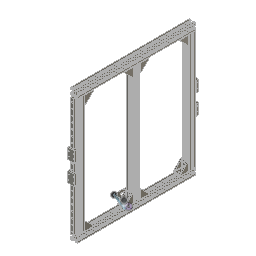
сборка станка вер 1.1.1 (Autodesk Fusion 360 design; units mm, degrees)
Autodesk Fusion 360 part; units mm, degrees
sketch "Sketch1" plane through (0, 0, 0) normal (0, 1, 0) x (1, 0, 0)
  line L0 (6.0101, -7) -> (-6.0101, -7)
  line L1 (-8.1, -12.8) -> (-8.1, -9.0899)
  line L2 (-6.0101, -7) -> (-8.1, -9.0899)
  line L3 (-4.1, -14.2) -> (-4.9, -14.2)
  line L4 (-4.9, -14.2) -> (-4.9, -15)
  line L5 (-4.1, -14.2) -> (-4.1, -12.8)
  line L6 (-13, -15) -> (-4.9, -15)
  line L7 (-8.1, -12.8) -> (-4.1, -12.8)
  line L8 (6.0101, -7) -> (8.1, -9.0899)
  line L9 (8.1, -12.8) -> (8.1, -9.0899)
  line L10 (8.1, -12.8) -> (4.1, -12.8)
  line L11 (4.1, -14.2) -> (4.1, -12.8)
  line L12 (4.1, -14.2) -> (4.9, -14.2)
  line L13 (4.9, -14.2) -> (4.9, -15)
  line L14 (13, -15) -> (4.9, -15)
  line L15 (14.2, -4.1) -> (14.2, -4.9)
  line L16 (12.8, -8.1) -> (9.0899, -8.1)
  line L17 (15, -13) -> (15, -4.9)
  line L18 (7, 6.0101) -> (9.0899, 8.1)
  line L19 (7, 6.0101) -> (7, -6.0101)
  line L20 (14.2, 4.9) -> (15, 4.9)
  line L21 (7, -6.0101) -> (9.0899, -8.1)
  line L22 (14.2, -4.1) -> (12.8, -4.1)
  line L23 (14.2, 4.1) -> (12.8, 4.1)
  line L24 (15, 13) -> (15, 4.9)
  line L25 (14.2, -4.9) -> (15, -4.9)
  line L26 (12.8, 8.1) -> (9.0899, 8.1)
  line L27 (12.8, 8.1) -> (12.8, 4.1)
  line L28 (12.8, -8.1) -> (12.8, -4.1)
  line L29 (14.2, 4.1) -> (14.2, 4.9)
  line L30 (4.1, 14.2) -> (4.9, 14.2)
  line L31 (8.1, 12.8) -> (8.1, 9.0899)
  line L32 (13, 15) -> (4.9, 15)
  line L33 (-6.0101, 7) -> (-8.1, 9.0899)
  line L34 (-6.0101, 7) -> (6.0101, 7)
  line L35 (-4.9, 14.2) -> (-4.9, 15)
  line L36 (6.0101, 7) -> (8.1, 9.0899)
  line L37 (4.1, 14.2) -> (4.1, 12.8)
  line L38 (-4.1, 14.2) -> (-4.1, 12.8)
  line L39 (-13, 15) -> (-4.9, 15)
  line L40 (4.9, 14.2) -> (4.9, 15)
  line L41 (-8.1, 12.8) -> (-8.1, 9.0899)
  line L42 (-8.1, 12.8) -> (-4.1, 12.8)
  line L43 (8.1, 12.8) -> (4.1, 12.8)
  line L44 (-4.1, 14.2) -> (-4.9, 14.2)
  line L45 (-14.2, 4.1) -> (-14.2, 4.9)
  line L46 (-12.8, 8.1) -> (-9.0899, 8.1)
  line L47 (-15, 13) -> (-15, 4.9)
  line L48 (-7, -6.0101) -> (-9.0899, -8.1)
  line L49 (-7, -6.0101) -> (-7, 6.0101)
  line L50 (-14.2, -4.9) -> (-15, -4.9)
  line L51 (-7, 6.0101) -> (-9.0899, 8.1)
  line L52 (-14.2, 4.1) -> (-12.8, 4.1)
  line L53 (-14.2, -4.1) -> (-12.8, -4.1)
  line L54 (-15, -13) -> (-15, -4.9)
  line L55 (-14.2, 4.9) -> (-15, 4.9)
  line L56 (-12.8, -8.1) -> (-9.0899, -8.1)
  line L57 (-12.8, -8.1) -> (-12.8, -4.1)
  line L58 (-12.8, 8.1) -> (-12.8, 4.1)
  line L59 (-14.2, -4.1) -> (-14.2, -4.9)
  circle A0 centre (0, 0) radius 5
  circle A1 centre (-11.55, -11.55) radius 2.25
  circle A2 centre (11.55, -11.55) radius 2.25
  circle A3 centre (11.55, 11.55) radius 2.25
  circle A4 centre (-11.55, 11.55) radius 2.25
  arc A5 (-15, -13) -> (-13, -15) centre (-13, -13) ccw
  arc A6 (13, -15) -> (15, -13) centre (13, -13) ccw
  arc A7 (15, 13) -> (13, 15) centre (13, 13) ccw
  arc A8 (-13, 15) -> (-15, 13) centre (-13, 13) ccw
  dimension "d17" = 10
  dimension "d22" = 4.5
  dimension "d24" = 360
  dimension "d25" = 2
  constraint coincident A0.centre origin
  constraint tangent L54 A5
  constraint tangent L6 A5
  constraint tangent L14 A6
  constraint tangent L17 A6
  constraint equal A5 A6
  constraint tangent L24 A7
  constraint tangent L32 A7
  constraint equal A5 A7
  constraint tangent L39 A8
  constraint tangent L47 A8
  constraint equal A5 A8
  measures "d17" diameter of A0
  measures "d22" diameter of A1
  measures "d25" radius of A5
extrude "Extrude1" add sketch "Sketch1" along normal blind 500 makes body 1
sketch "Sketch3" plane through (15, 0, 0) normal (1, 0, 0) x (0, 1, 0)
  line L0 (0, 13) -> (0, 4.9)
  line L1 (0, 4.9) -> (500, 4.9)
  line L2 (500, 4.9) -> (500, 13)
  line L3 (500, 13) -> (0, 13)
  line L4 (0, 15) -> (35, 15)
  line L5 (35, 15) -> (35, 19)
  line L6 (4, 50) -> (0, 50)
  line L7 (0, 50) -> (0, 15)
  line L8 (4, 50) -> (35, 19)
  line L9 (4, 50) -> (4, 19)
  line L10 (35, 19) -> (4, 19)
  dimension "d35" = 35
  dimension "d36" = 35
  dimension "d38" = 4
  dimension "d39" = 4
  dimension "d40" = 4
  constraint horizontal L4
  constraint vertical L5
  constraint horizontal L6
  constraint vertical L7
  constraint perpendicular L4 L9
  constraint perpendicular L9 L10
  measures "d35" distance of L4.start L4.end
  measures "d36" distance of L4.start L6.end
  measures "d38" distance of L6.end L6.start
  measures "d39" distance of L4.end L5.end
  measures "d40" distance of L7 L9
extrude "Extrude2" add sketch "Sketch3" against normal blind 30 separate body contours L4 L5 L6 L7 L9 L10 makes body 2
extrude "Extrude3" add sketch "Sketch3" against normal blind 4 contours L8 L9 L10 bodies 2 1
extrude "Extrude4" add sketch "Sketch3" along normal blind -26 and the other way blind 30 contours L8 L9 L10 bodies 1 2
sketch "Sketch4" plane through (0, 0, 19) normal (0, 0, 1) x (-1, 0, 0)
  line L0 (11, -35) -> (11, -4)
  line L1 (11, -4) -> (-11, -4)
  line L2 (-11, -4) -> (-11, -35)
  line L3 (-11, -35) -> (11, -35)
  line L4 (-11, -4) -> (-9, -4)
  circle A0 centre (0, -12.25) radius 3
  circle A1 centre (0, -27.25) radius 3
  point P0 (0, -35)
  dimension "d51" = 6
  dimension "d52" = 6
  constraint coincident L1.end L2.start
  constraint coincident L1 L4.end
  measures "d51" diameter of A0
  measures "d52" diameter of A1
extrude "Extrude5" cut sketch "Sketch4" against normal blind 8 contours A0 | A1 bodies 2 1
sketch "Sketch5" plane through (0, 4, 0) normal (0, 1, 0) x (-1, 0, 0)
  line L0 (11, 19) -> (11, 50)
  line L1 (11, 50) -> (-11, 50)
  line L2 (-11, 50) -> (-11, 19)
  line L3 (-11, 19) -> (11, 19)
  circle A0 centre (0, 41.75) radius 3
  circle A1 centre (0, 26.75) radius 3
  dimension "d57" = 6
  dimension "d58" = 6
  measures "d57" diameter of A0
  measures "d58" diameter of A1
extrude "Extrude6" cut sketch "Sketch5" against normal blind 6 contours A0 | A1 bodies 2
fillet "Fillet1" radius 3 1 edges at (0, 4, 19) on bodies 2
fillet "Fillet2" radius 2 6 edges at (11, 4, 36) (11, 4.8787, 19.8787) (11, 21, 19) (-11, 21, 19) (-11, 4.8787, 19.8787) (-11, 4, 36) on bodies 2
copy_body "Body->Comp1" bodies 2 removing the originals makes body 3 in component "уголок 30 2хМ6"
copy_body "Body->Comp2" bodies 1 removing the originals makes body 4 in component "профиль 3030 500mm"
move_body "Move1" bodies 3 to x (1, 0, 0) y (0, 1, 0) z (0, 0, 1) at (0, 30, 0) in component "уголок 30 2хМ6"
sketch "Sketch6" plane through (0, 0, 515) normal (0, 0, 1) x (-1, 0, 0)
  circle A0 centre (-11.55, -3.45) radius 2.25
  circle A1 centre (-11.55, -26.55) radius 2.25
  circle A2 centre (11.55, -26.55) radius 2.25
  circle A3 centre (11.55, -3.45) radius 2.25
  circle A4 centre (0, -15) radius 5
  line L0 (4.9, -0.8) -> (4.1, -0.8)
  line L1 (4.1, -0.8) -> (4.1, -2.2)
  line L2 (4.1, -2.2) -> (8.1, -2.2)
  line L3 (8.1, -2.2) -> (8.1, -5.9101)
  line L4 (8.1, -5.9101) -> (6.0101, -8)
  line L5 (6.0101, -8) -> (-6.0101, -8)
  line L6 (-6.0101, -8) -> (-8.1, -5.9101)
  line L7 (-8.1, -5.9101) -> (-8.1, -2.2)
  line L8 (-8.1, -2.2) -> (-4.1, -2.2)
  line L9 (-4.1, -2.2) -> (-4.1, -0.8)
  line L10 (-4.1, -0.8) -> (-4.9, -0.8)
  line L11 (-4.9, -0.8) -> (-4.9, 0)
  line L12 (-4.9, 0) -> (-13, 0)
  arc A5 (-13, 0) -> (-15, -2) centre (-13, -2) ccw
  line L13 (-15, -2) -> (-15, -10.1)
  line L14 (-15, -10.1) -> (-14.2, -10.1)
  line L15 (-14.2, -10.1) -> (-14.2, -10.9)
  line L16 (-14.2, -10.9) -> (-12.8, -10.9)
  line L17 (-12.8, -10.9) -> (-12.8, -6.9)
  line L18 (-12.8, -6.9) -> (-9.0899, -6.9)
  line L19 (-9.0899, -6.9) -> (-7, -8.9899)
  line L20 (-7, -8.9899) -> (-7, -21.0101)
  line L21 (-7, -21.0101) -> (-9.0899, -23.1)
  line L22 (-9.0899, -23.1) -> (-12.8, -23.1)
  line L23 (-12.8, -23.1) -> (-12.8, -19.1)
  line L24 (-12.8, -19.1) -> (-14.2, -19.1)
  line L25 (-14.2, -19.1) -> (-14.2, -19.9)
  line L26 (-14.2, -19.9) -> (-15, -19.9)
  line L27 (-15, -19.9) -> (-15, -28)
  arc A6 (-15, -28) -> (-13, -30) centre (-13, -28) ccw
  line L28 (-13, -30) -> (-4.9, -30)
  line L29 (-4.9, -30) -> (-4.9, -29.2)
  line L30 (-4.9, -29.2) -> (-4.1, -29.2)
  line L31 (-4.1, -29.2) -> (-4.1, -27.8)
  line L32 (-4.1, -27.8) -> (-8.1, -27.8)
  line L33 (-8.1, -27.8) -> (-8.1, -24.0899)
  line L34 (-8.1, -24.0899) -> (-6.0101, -22)
  line L35 (-6.0101, -22) -> (6.0101, -22)
  line L36 (6.0101, -22) -> (8.1, -24.0899)
  line L37 (8.1, -24.0899) -> (8.1, -27.8)
  line L38 (8.1, -27.8) -> (4.1, -27.8)
  line L39 (4.1, -27.8) -> (4.1, -29.2)
  line L40 (4.1, -29.2) -> (4.9, -29.2)
  line L41 (4.9, -29.2) -> (4.9, -30)
  line L42 (4.9, -30) -> (13, -30)
  arc A7 (13, -30) -> (15, -28) centre (13, -28) ccw
  line L43 (15, -28) -> (15, -19.9)
  line L44 (15, -19.9) -> (14.2, -19.9)
  line L45 (14.2, -19.9) -> (14.2, -19.1)
  line L46 (14.2, -19.1) -> (12.8, -19.1)
  line L47 (12.8, -19.1) -> (12.8, -23.1)
  line L48 (12.8, -23.1) -> (9.0899, -23.1)
  line L49 (9.0899, -23.1) -> (7, -21.0101)
  line L50 (7, -21.0101) -> (7, -8.9899)
  line L51 (7, -8.9899) -> (9.0899, -6.9)
  line L52 (9.0899, -6.9) -> (12.8, -6.9)
  line L53 (12.8, -6.9) -> (12.8, -10.9)
  line L54 (12.8, -10.9) -> (14.2, -10.9)
  line L55 (14.2, -10.9) -> (14.2, -10.1)
  line L56 (14.2, -10.1) -> (15, -10.1)
  line L57 (15, -10.1) -> (15, -2)
  arc A8 (15, -2) -> (13, 0) centre (13, -2) ccw
  line L58 (13, 0) -> (4.9, 0)
  line L59 (4.9, 0) -> (4.9, -0.8)
  line L60 (0, 13) -> (13.5, 13)
  line L61 (13.5, 13) -> (13.5, 3)
  line L62 (6, 3) -> (13.5, 3)
  line L63 (6, 3) -> (6, 0)
  line L64 (0, 0) -> (6, 0)
  line L65 (-6, 3) -> (-6, 0)
  line L66 (-6, 3) -> (-13.5, 3)
  line L67 (-4.9, 0) -> (-4.9, -0.8)
  line L68 (-13.5, 13) -> (-13.5, 3)
  line L69 (-4.9, -0.8) -> (-4.1, -0.8)
  line L70 (0, 0) -> (-6, 0)
  line L71 (0, 13) -> (-13.5, 13)
  line L72 (0, 8) -> (6, 8)
  line L73 (6, 8) -> (6, 3)
  line L74 (0, 8) -> (-6, 8)
  line L75 (-6, 8) -> (-6, 3)
  point P0 (-13, 0)
  dimension "d65" = 13.5
  constraint coincident L64.start L70.start
  constraint perpendicular L60 L61
  constraint perpendicular L61 L62
  constraint coincident L58 L63.end
  constraint perpendicular L58 L63
  constraint perpendicular L63 L64
  measures "d65" distance of L60.start L60.end
extrude "Extrude1'" add sketch "Sketch6" against normal blind 500 separate body contours L12 L58 L63 L64 L65 L70 L72 L73 L74 L75 makes body 5 in component "направляющая 500мм 2 каретки"
sketch "Sketch7" plane through (0, -8, 0) normal (0, -1, 0) x (1, 0, 0)
  line L0 (6, 515) -> (-6, 515)
  line L1 (-6, 515) -> (-6, 15)
  line L2 (-6, 15) -> (6, 15)
  line L3 (6, 15) -> (6, 515)
  circle A0 centre (0, 25) radius 1.75
  circle A1 centre (0, 25) radius 3
  line L4 (0, 25) -> (0, 26.75)
  circle A2 centre (0, 50) radius 3
  circle A3 centre (0, 50) radius 1.75
  circle A4 centre (0, 75) radius 3
  circle A5 centre (0, 75) radius 1.75
  circle A6 centre (0, 100) radius 3
  circle A7 centre (0, 100) radius 1.75
  circle A8 centre (0, 125) radius 3
  circle A9 centre (0, 125) radius 1.75
  circle A10 centre (0, 150) radius 3
  circle A11 centre (0, 150) radius 1.75
  circle A12 centre (0, 175) radius 3
  circle A13 centre (0, 175) radius 1.75
  circle A14 centre (0, 200) radius 3
  circle A15 centre (0, 200) radius 1.75
  circle A16 centre (0, 225) radius 3
  circle A17 centre (0, 225) radius 1.75
  circle A18 centre (0, 250) radius 3
  circle A19 centre (0, 250) radius 1.75
  circle A20 centre (0, 275) radius 3
  circle A21 centre (0, 275) radius 1.75
  circle A22 centre (0, 300) radius 3
  circle A23 centre (0, 300) radius 1.75
  circle A24 centre (0, 325) radius 3
  circle A25 centre (0, 325) radius 1.75
  circle A26 centre (0, 350) radius 3
  circle A27 centre (0, 350) radius 1.75
  circle A28 centre (0, 375) radius 3
  circle A29 centre (0, 375) radius 1.75
  circle A30 centre (0, 400) radius 3
  circle A31 centre (0, 400) radius 1.75
  circle A32 centre (0, 425) radius 3
  circle A33 centre (0, 425) radius 1.75
  circle A34 centre (0, 450) radius 3
  circle A35 centre (0, 450) radius 1.75
  circle A36 centre (0, 475) radius 3
  circle A37 centre (0, 475) radius 1.75
  circle A38 centre (0, 500) radius 3
  circle A39 centre (0, 500) radius 1.75
  dimension "d68" = 3.5
  dimension "d71" = 0
  dimension "d72" = 475
  constraint concentric A0 A1
  constraint coincident A0.centre A1.centre
  constraint coincident A0 L4.end
  constraint vertical L4
  measures "d68" diameter of A0
extrude "Extrude2'" cut sketch "Sketch7" against normal blind 10 contours A0 | A3 | A5 | A7 | A9 | A11 | A13 | A15 | A17 | A19 | A21 | A23 | A25 | A27 | A29 | A31 | A33 | A35 | A37 | A39 bodies 5 in component "направляющая 500мм 2 каретки"
extrude "Extrude3'" cut sketch "Sketch7" against normal blind 4.5 contours A1 | A2 | A4 | A6 | A8 | A10 | A12 | A14 | A16 | A18 | A20 | A22 | A24 | A26 | A28 | A30 | A32 | A34 | A36 | A38 bodies 5 in component "направляющая 500мм 2 каретки"
extrude "Extrude4'" add sketch "Sketch6" along normal blind -270 and the other way blind 315.4 contours L60 L61 L62 L66 L68 L71 L72 L73 L74 L75 bodies 5 in component "направляющая 500мм 2 каретки"
extrude "Extrude5'" add sketch "Sketch6" along normal blind -230 and the other way blind 184.6 contours L60 L61 L62 L66 L68 L71 L72 L73 L74 L75 bodies 5 in component "направляющая 500мм 2 каретки"
sketch "Sketch9" plane through (0, -13, 0) normal (0, -1, 0) x (1, 0, 0)
  line L0 (13.5, 245) -> (-13.5, 245)
  line L1 (-13.5, 245) -> (-13.5, 199.6)
  line L2 (-13.5, 199.6) -> (13.5, 199.6)
  line L3 (13.5, 199.6) -> (13.5, 245)
  circle A0 centre (10, 212.3) radius 1.5
  circle A1 centre (-10, 212.3) radius 1.5
  circle A2 centre (10, 232.3) radius 1.5
  circle A3 centre (-10, 232.3) radius 1.5
  line L4 (0, 245) -> (0, 285)
  line L5 (0, 265) -> (13, 265)
  circle A4 centre (10, 317.7) radius 1.5
  circle A5 centre (-10, 317.7) radius 1.5
  circle A6 centre (-10, 297.7) radius 1.5
  circle A7 centre (10, 297.7) radius 1.5
  point P0 (0, 222.3)
  dimension "d85" = 20
  dimension "d86" = 20
  dimension "d87" = 3
  dimension "d88" = 3
  dimension "d89" = 3
  dimension "d90" = 3
  constraint midpoint L0 L4.start
  constraint perpendicular L0 L4
  constraint midpoint L4 L5.start
  constraint perpendicular L4 L5
  constraint symmetric A0 L5 A4
  constraint symmetric A1 L5 A5
  constraint symmetric A2 L5 A7
  constraint symmetric A3 L5 A6
  measures "d85" distance of A0.centre A1.centre
  measures "d86" distance of A0.centre A2.centre
  measures "d87" diameter of A0
  measures "d88" diameter of A1
  measures "d89" diameter of A2
  measures "d90" diameter of A3
extrude "Extrude6'" cut sketch "Sketch9" against normal blind 3.5 contours A0 | A1 | A2 | A3 | A4 | A5 | A6 | A7 bodies 5 in component "направляющая 500мм 2 каретки"
sketch "Sketch10" plane through (0, 0, -15) normal (0, 0, -1) x (1, 0, 0)
  line L0 (-4.9, 0) -> (-13, 0)
  line L1 (-13, 0) -> (-13, -500)
  line L2 (-13, -500) -> (-4.9, -500)
  line L3 (-4.9, -500) -> (-4.9, 0)
  line L4 (-13, -500) -> (-13, 0)
  line L5 (-60, -250) -> (-60, -229)
  line L6 (-60, -229) -> (-18, -229)
  line L7 (-18, -229) -> (-18, -250)
  circle A0 centre (-54.75, -234.25) radius 1.5
  circle A1 centre (-23.25, -234.25) radius 1.5
  arc A2 (-28, -250) -> (-50, -250) centre (-39, -250) ccw
  line L8 (-18, -271) -> (-18, -250)
  line L9 (-60, -271) -> (-18, -271)
  line L10 (-60, -250) -> (-60, -271)
  circle A3 centre (-54.75, -265.75) radius 1.5
  circle A4 centre (-23.25, -265.75) radius 1.5
  arc A5 (-50, -250) -> (-28, -250) centre (-39, -250) ccw
  circle A6 centre (-39, -250) radius 2.5
  point P0 (-39, -250)
  dimension "d95" = 42
  dimension "d98" = 3
  dimension "d99" = 3
  dimension "d100" = 22
  dimension "d101" = 5
  constraint coincident L1.end L2.start
  constraint coincident L0.end L1.start
  constraint perpendicular L5 L6
  constraint coincident P0 A2.centre
  constraint concentric A2 A6
  measures "d95" distance of L7.end L5.start
  measures "d98" diameter of A0
  measures "d99" diameter of A1
  measures "d100" diameter of A2
  measures "d101" diameter of A6
sketch "Sketch11" plane through (0, 229, 0) normal (0, -1, 0) x (1, 0, 0)
  line L0 (-60, 12) -> (-18, 12)
  line L1 (-18, 12) -> (-18, 15)
  line L2 (-18, 15) -> (-60, 15)
  line L3 (-60, 15) -> (-60, 12)
  line L4 (-18, 12) -> (-18, -15.0433)
  line L5 (-18, -15.0433) -> (-17.9922, -15.0433)
  line L6 (-17.9922, -15.0433) -> (-17.9922, 12)
  line L7 (-17.9922, -15.0433) -> (-60, 12)
  line L8 (-18, 15) -> (-15, 15)
  line L9 (-15, 15) -> (-15, -15)
  line L10 (-15, -15) -> (-18, -15)
  line L11 (-18, -15) -> (-18, 15)
  line L12 (-16, 0) -> (0, 0)
  constraint coincident L0.end L1.start
  constraint perpendicular L0 L4
  constraint perpendicular L4 L5
  constraint coincident L0 L6.end
  constraint perpendicular L0 L6
  constraint coincident L0.start L3.end
  constraint horizontal L8
  constraint vertical L9
  constraint horizontal L10
  constraint vertical L11
  constraint coincident L1.end L2.start
  constraint coincident L12.end origin
  constraint perpendicular L9 L12
extrude "Extrude7" add sketch "Sketch10" along normal blind -30 and the other way blind 27 separate body contours L5 L6 L7 L8 L9 L10 makes body 6
extrude "Extrude9" add sketch "Sketch11" along normal blind -42 and the other way blind 46 contours L0 L1 L2 L3 L11 | L0 L4 L7 L11 | L1 L4 L8 L9 L10 L11 bodies 6
extrude "Extrude8" add sketch "Sketch11" along normal blind 4 contours L0 L1 L2 L3 L11 | L0 L4 L7 L11 | L1 L4 L8 L9 L10 L11 bodies 6
extrude "Extrude10" add sketch "Sketch11" against normal blind 46 contours L1 L4 L8 L9 L10 L11 bodies 6
component "уголок 30 2хМ6" placed x (1, 0, 0) y (0, 1, 0) z (0, 0, 1) at (0, 0, 0)
component "профиль 3030 500mm" placed x (1, 0, 0) y (0, 1, 0) z (0, 0, 1) at (0, 0, 0)
component "профиль 3030 500mm" placed x (1, 0, 0) y (0, 0, -1) z (0, 1, 0) at (0, 485, 515)
component "профиль 3030 500mm" placed x (1, 0, 0) y (0, 0, -1) z (0, 1, 0) at (0, 15, 515)
component "уголок 30 2хМ6" placed x (1, 0, 0) y (0, 0, -1) z (0, 1, 0) at (0, 15.0029, 544.249)
component "уголок 30 2хМ6" placed x (1, 0, 0) y (0, 0, -1) z (0, 1, 0) at (0, 250.0029, 544.249)
component "уголок 30 2хМ6" placed x (1, 0, 0) y (0, 1, 0) z (0, 0, 1) at (0, 235, 0)
component "уголок 30 2хМ6" placed x (1, 0, 0) y (0, 0, 1) z (0, -1, 0) at (0, 249.249, -15.0029)
component "уголок 30 2хМ6" placed x (1, 0, 0) y (0, -1, 0) z (0, 0, -1) at (0, 264.252, 529.2461)
component "уголок 30 2хМ6" placed x (1, 0, 0) y (0, -1, 0) z (0, 0, -1) at (0, 499.252, 529.2461)
component "уголок 30 2хМ6" placed x (1, 0, 0) y (0, 0, 1) z (0, -1, 0) at (0, 484.249, -15.0029)
component "профиль 3030 500mm" placed x (1, 0, 0) y (0, 1, 0) z (0, 0, 1) at (0, 0, 530)
component "направляющая 500мм 2 каретки" placed x (1, 0, 0) y (0, 1, 0) z (0, 0, 1) at (0, 0, 0)
component "профиль 3030 500mm" placed x (1, 0, 0) y (0, 0, -1) z (0, 1, 0) at (0, 250, 515)
component "направляющая 500мм 2 каретки" placed x (-1, 0, 0) y (0, -1, 0) z (0, 0, 1) at (0, 499.9207, 0)
